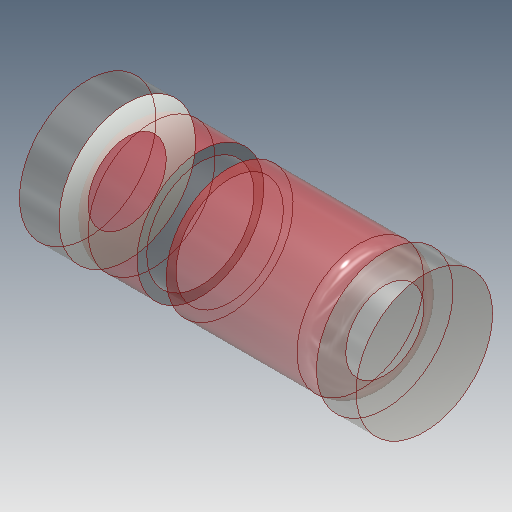
# Autodesk Inventor part: sod-80
Saved by Autodesk Inventor 2017 (Build 210142000, 142)
## iProperties
Created: 2016-03-02
Part Number: sod-80
Material: Glass
Document SubType Name: Modeling
Designer: Sawaiz
Density: 2.18 g/cm^3
Appearance: Dark Red
Author: Sawaiz
Autodesk Inventor part; units mm, degrees
ref_plane "YZ Plane" through (0, 0, 0) normal (1, 0, 0) x (0, 1, 0)
ref_plane "XZ Plane" through (0, 0, 0) normal (0, 1, 0) x (-1, 0, 0)
ref_plane "XY Plane" through (0, 0, 0) normal (0, 0, 1) x (1, 0, 0)
sketch "Sketch1" plane through (0, 0, 0) normal (0, 1, 0) x (-1, 0, 0)
  circle A0 centre (0, 0) radius 0.7
  dimension "d0" = 1.4
  constraints: 1 centre point, 1 coincident
  measures "d0" diameter of A0
extrude "Extrusion1" add sketch "Sketch1" along normal mid plane 3.45
sketch "Sketch2" plane through (0, 0, 0) normal (1, 0, 0) x (0, 1, 0)
  line L0 (-1.725, 0.7) -> (-1.725, -0.7) projected
  line L1 (1.725, -0.7) -> (1.725, 0.7) projected
  line L2 (-1.32, 0.7) -> (-1.32, 0.4)
  line L3 (-1.725, 0.7) -> (1.725, 0.7) projected
  arc A0 (-1.07, 0.65) -> (-1.32, 0.4) centre (-1.07, 0.4) ccw
  line L4 (-1.07, 0.65) -> (0, 0.65)
  line L5 (0, 0.65) -> (0, 0.7)
  line L6 (-2.415, 0) -> (2.415, 0) projected
  point P0 (0, 0)
  dimension "d3" = 1.32
  dimension "d5" = 0.65
  dimension "d6" = 0.25
  constraints: 6 end point, 2 point on circle, 2 tangent, 1 centre point, 1 horizontal, 1 midpoint, 1 vertical
  measures "d3" distance from line of L2 point (0, 0)
  measures "d5" distance from line of point (0, 0) L4
  measures "d6" radius of A0
revolve "Revolution1" cut sketch "Sketch2" angle 360 about axis through (0, -10, 0) along (0, 1, 0) fills toward (-0.005, 0.675) open curves L5 L4 A0 L2
mirror "Mirror1" about plane through (0, 0, 0) normal (0, 1, 0) of "Revolution1"
sketch "Sketch3" plane through (0, 0, 0) normal (1, 0, 0) x (0, 1, 0)
  line L0 (1.07, 0.65) -> (1.07, -0.65) projected
  line L1 (-1.07, 0.65) -> (-1.07, -0.65) projected
  line L2 (-1.07, 0.65) -> (1.07, 0.65) projected
  line L3 (-0.57, 0.65) -> (-0.27, 0.65)
  line L4 (-0.27, 0.65) -> (-0.27, 0.55)
  line L5 (-0.27, 0.55) -> (-0.57, 0.55)
  line L6 (-0.57, 0.55) -> (-0.57, 0.65)
  line L7 (-2.415, 0) -> (2.415, 0) projected
  point P0 (0, 0)
  dimension "d9" = 0.3
  dimension "d10" = 0.1
  dimension "d11" = 0.5
  constraints: 8 end point, 2 parallel, 1 horizontal, 1 perpendicular, 1 point on line
  measures "d9" distance of L4.end L5.end
  measures "d10" distance of L5.end L3.start
  measures "d11" distance between parallel lines of L1 L6
revolve "Revolution2" cut sketch "Sketch3" angle 360 about axis through (0, -10, 0) along (0, 1, 0) contours L4 L5 L6 L2
body "Solid1"
